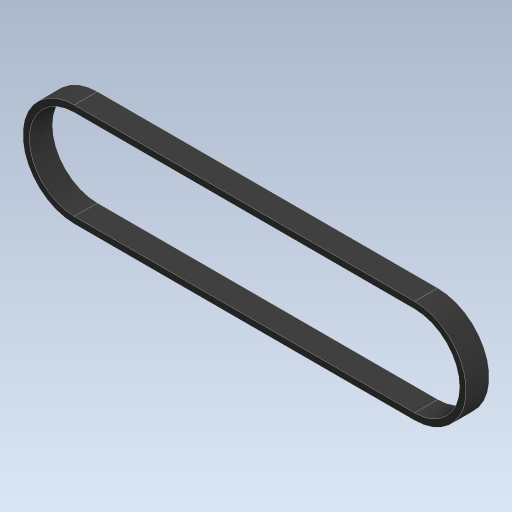
# Autodesk Inventor part: INDX_019_FeederBelt
Saved by Autodesk Inventor 2024 (Build 280153000, 153)
## iProperties
Created: 2024-08-09
Part Number: INDX_019_FeederBelt
Material: Rubber
Document SubType Name: Modeling
Designer: Oscar
Density: 0.93 g/cm^3
Appearance: Rubber - Black
Author: Oscar
Autodesk Inventor part; units mm, degrees
ref_plane "YZ Plane" through (0, 0, 0) normal (1, 0, 0) x (0, 1, 0)
ref_plane "XZ Plane" through (0, 0, 0) normal (0, 1, 0) x (-1, 0, 0)
ref_plane "XY Plane" through (0, 0, 0) normal (0, 0, 1) x (1, 0, 0)
sketch "Sketch1" plane through (0, 0, 0) normal (0, 0, 1) x (1, 0, 0)
  arc A0 (0, 17.5133) -> (0, -17.5133) centre (0, 0) ccw
  arc A1 (132.5118, -17.5133) -> (132.5118, 17.5133) centre (132.5118, 0) ccw
  line L0 (0, 17.5133) -> (132.5118, 17.5133)
  line L1 (0, -17.5133) -> (132.5118, -17.5133)
  arc A2 (132.5118, -20.0533) -> (132.5118, 20.0533) centre (132.5118, 0) ccw
  line L2 (132.5118, -20.0533) -> (0, -20.0533)
  arc A3 (0, 20.0533) -> (0, -20.0533) centre (0, 0) ccw
  line L3 (0, 20.0533) -> (132.5118, 20.0533)
  dimension "d0" = 35.0266
  dimension "d1" = 132.5118
  dimension "d2" = 2.54
  constraints: 9 end point, 8 point on circle, 4 centre point, 2 parallel, 2 tangent, 1 coincident, 1 equal radius, 1 horizontal alignment, 3 other
  measures "d0" diameter of A0
  measures "d1" distance of A1.centre A0.centre
  measures "d2" distance between parallel lines of L0 L3
extrude "Extrusion1" add sketch "Sketch1" along normal blind 9
body "Solid1"
